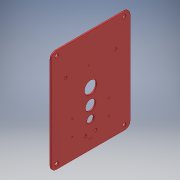
# Autodesk Inventor part: +XPanel_PCB
Saved by Autodesk Inventor 2018 (Build 220112000, 112)
## iProperties
Created: 2018-07-05
Part Number: +XPanel_PCB
Material: Epoxy Resin
Document SubType Name: Modeling
Designer: Bradley
Density: 1.14 g/cm^3
Appearance: Smooth - Red
Mass: 8.24144 g
Surface Area: 149.532 cm^2
Volume: 7.22933 cm^3
Author: Bradley
Autodesk Inventor part; units mm, degrees
ref_plane "YZ Plane" through (0, 0, 0) normal (1, 0, 0) x (0, 1, 0)
ref_plane "XZ Plane" through (0, 0, 0) normal (0, 1, 0) x (-1, 0, 0)
ref_plane "XY Plane" through (0, 0, 0) normal (0, 0, 1) x (1, 0, 0)
sketch "Sketch1" plane through (0, 0, 0) normal (1, 0, 0) x (0, 1, 0)
  line L0 (-33, -49.5) -> (33, -49.5)
  line L1 (38, -44.5) -> (38, 44.5)
  line L2 (33, 49.5) -> (-33, 49.5)
  line L3 (-38, 44.5) -> (-38, -44.5)
  line L4 (-38, -49.5) -> (38, 49.5) construction
  line L5 (38, -49.5) -> (-38, 49.5) construction
  arc A0 (-33, 49.5) -> (-38, 44.5) centre (-33, 44.5) ccw
  arc A1 (38, 44.5) -> (33, 49.5) centre (33, 44.5) ccw
  arc A2 (33, -49.5) -> (38, -44.5) centre (33, -44.5) ccw
  arc A3 (-38, -44.5) -> (-33, -49.5) centre (-33, -44.5) ccw
  point P0 (0, 0)
  dimension "d0" = 76
  dimension "d1" = 99
  dimension "d2" = 5
  constraints: 12 end point, 8 point on circle, 8 point on line, 8 tangent, 4 centre point, 3 equal radius, 2 midpoint, 2 parallel, 1 horizontal, 1 perpendicular
  measures "d0" distance of L4.end L5.end
  measures "d1" distance of L5.end L4.start
  measures "d2" radius of A0
extrude "Extrusion1" add sketch "Sketch1" along normal mid plane 1
sketch "Sketch2" plane through (0.5, 0, 0) normal (1, 0, 0) x (0, 0, -1)
  line L0 (45, -32.5) -> (-45, -32.5) construction
  line L1 (-45, -32.5) -> (-45, 32.5) construction
  line L2 (-45, 32.5) -> (45, 32.5) construction
  line L3 (45, 32.5) -> (45, -32.5) construction
  line L4 (45, -32.5) -> (-45, 32.5) construction
  line L5 (-45, -32.5) -> (45, 32.5) construction
  point P0 (0, 0)
  dimension "d5" = 90
  dimension "d6" = 65
  constraints: 12 end point, 4 coincident, 2 midpoint, 2 parallel, 1 horizontal, 1 perpendicular
  measures "d5" distance of L1.end L2.end
  measures "d6" distance of L0.end L1.end
hole "Hole1" at (0.5, -32.5, 45) at (0.5, 32.5, 45) at (0.5, 32.5, -45) at (0.5, -32.5, -45) direction (-1, 0, 0) diameter 3.3 end through all
sketch "Sketch3" plane through (0.5, 0, 0) normal (1, 0, 0) x (0, 0, -1)
  circle A0 centre (-2.5, 0) radius 6
  circle A1 centre (12.35, 0) radius 5
  circle A2 centre (-21.5, -1.75) radius 0.475
  circle A3 centre (24, 0) radius 3.5
  circle A4 centre (40, 1) radius 0.3
  circle A5 centre (40, -1) radius 0.3
  line L0 (40, -1) -> (40, 1) construction
  line L1 (40, 1) -> (40, 5.4827) construction
  ellipse E0 centre (0, 0) end of major axis (40.5, 0) minor radius 35 construction
  line L2 (35.5, -5) -> (35.5, 5) construction
  circle A6 centre (35.5, -5) radius 4.511 construction
  ellipse E1 centre (0, 0) end of major axis (35.989, 0) minor radius 30.489 construction
  line L3 (-22.384, -23.8741) -> (-22.384, 23.8741) construction
  line L4 (-2.5, 0) -> (-37.3972, 41.9) construction
  line L5 (-40, 41.9) -> (-5.1028, 0) construction
  line L6 (15, -17.5) -> (30, -17.5) construction
  line L7 (30, -17.5) -> (30, 17.5) construction
  line L8 (30, 17.5) -> (15, 17.5) construction
  line L9 (15, 17.5) -> (15, -17.5) construction
  circle A7 centre (15, -17.5) radius 0.5
  circle A8 centre (30, -17.5) radius 0.5
  circle A9 centre (30, 17.5) radius 0.5
  circle A10 centre (15, 17.5) radius 0.5
  point P0 (40, 0)
  point P1 (35.5, 0)
  point P2 (30, 0)
  dimension "d31" = 35
  dimension "d32" = 40.5
  dimension "d43" = 30.489
  dimension "d44" = 35.989
  dimension "d14" = 14.85
  dimension "d15" = 12
  dimension "d16" = 10
  dimension "d19" = 2.5
  dimension "d20" = 21.5
  dimension "d21" = 1.75
  dimension "d22" = 0.95
  dimension "d23" = 7
  dimension "d24" = 26.5
  dimension "d25" = 0.6
  dimension "d26" = 2
  dimension "d27" = 40
  dimension "d28" = 4.4827
  dimension "d33" = 10
  dimension "d34" = 4.5
  dimension "d42" = 9.0221
  dimension "d45" = 40
  dimension "d46" = 2
  dimension "d47" = 41.9
  dimension "d48" = 22.384
  dimension "d49" = 15
  dimension "d50" = 1
  dimension "d51" = 35
  dimension "d52" = 15
  constraints: 20 end point, 11 centre point, 8 horizontal alignment, 6 coincident, 4 equal radius, 4 vertical, 3 midpoint, 3 parallel, 1 horizontal, 1 perpendicular, 1 point on line, 8 other
  measures "d14" distance of A1.centre point (-2.5, 0)
  measures "d15" diameter of A0
  measures "d16" diameter of A1
  measures "d19" distance of point (0, 0) point (-2.5, 0)
  measures "d20" horizontal distance of point (0, 0) A2.centre
  measures "d21" vertical distance of point (0, 0) A2.centre
  measures "d22" diameter of A2
  measures "d23" diameter of A3
  measures "d24" distance of A3.centre point (-2.5, 0)
  measures "d25" diameter of A4
  measures "d26" distance of L0.start L0.end
  measures "d27" distance from line of point (0, 0) L0
  measures "d28" distance of L0.end L1.end
  measures "d33" distance of L2.start L2.end
  measures "d34" distance between parallel lines of L0 L2
  measures "d42" diameter of A6
  measures "d45" horizontal distance of point (0, 0) L5.start
  measures "d46" distance between parallel lines of L4 L5
  measures "d47" vertical distance of L4.start L4.end
  measures "d48" distance from line of point (0, 0) L3
  measures "d49" distance of L8.end L7.end
  measures "d50" diameter of A7
  measures "d51" distance of L6.end L7.end
  measures "d52" distance from line of point (0, 0) L9
extrude "Extrusion2" cut sketch "Sketch3" against normal through all
sketch "Sketch4" plane through (0.5, 0, 0) normal (1, 0, 0) x (0, 0, -1)
  point P0 (0, 0)
  point P1 (35.5, -5)
  point P2 (35.5, 5)
  point P3 (-22.384, -23.8741)
  point P4 (-22.384, 23.8741)
hole "Hole2" at (0.5, -5, -35.5) at (0.5, 5, -35.5) at (0.5, -23.8741, 22.384) at (0.5, 23.8741, 22.384) direction (-1, 0, 0) diameter 2.2 end through all clearance for "Flat Head Machine Screw" size "M2" standard "Ansi Metric M Profile"
equation "\"d43\" = d31 - 0.5 * d42"
equation "\"d44\" = d32 - 0.5 * d42"
body "Solid1"
